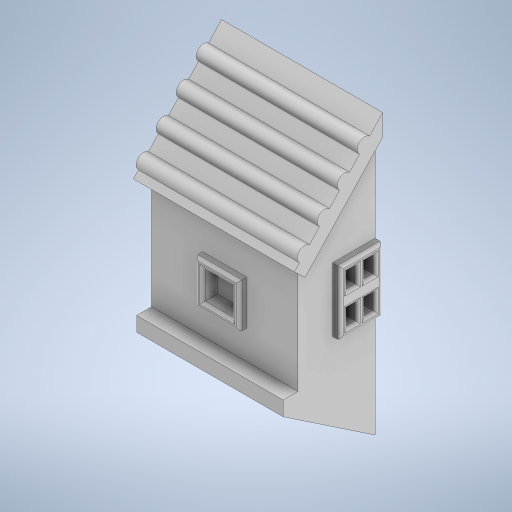
# Autodesk Inventor part: 背 物1
Saved by Autodesk Inventor 2024 (Build 280153000, 153)
## iProperties
Created: 2024-05-24
Part Number: 背 物1
Material: 一般
Document SubType Name: Modeling
Designer: User
Density: 1 g/cm^3
Appearance: 預設
Author: User
Autodesk Inventor part; units mm, degrees
ref_plane "YZ Plane" through (0, 0, 0) normal (1, 0, 0) x (0, 1, 0)
ref_plane "XZ Plane" through (0, 0, 0) normal (0, 1, 0) x (-1, 0, 0)
sketch "草圖1" plane through (0, 0, 0) normal (1, 0, 0) x (0, 1, 0)
  line L0 (0, 0) -> (7, 0)
  line L1 (7, 0) -> (7.6846, 0.7289)
  line L2 (7.6846, 0.7289) -> (14.0989, -5.2958)
  line L3 (0, 0) -> (0, 1)
  line L4 (0, 1) -> (-1, 1)
  line L5 (-1, 1) -> (-5.2258, -5.2958)
  line L6 (-5.2258, -5.2958) -> (14.0989, -5.2958)
  line L7 (7, 0) -> (12.6382, -5.2958)
  line L8 (2.0488, -5.2958) -> (6.4059, -5.2958)
  line L9 (6.4059, -5.2958) -> (6.4059, -2.3941)
  line L10 (6.4059, -2.3941) -> (2.0488, -2.3941)
  line L11 (2.0488, -2.3941) -> (2.0488, -5.2958)
  line L12 (5.9059, -2.8941) -> (4.7273, -2.8941)
  line L13 (4.7273, -2.8941) -> (4.7273, -3.5949)
  line L14 (4.7273, -3.5949) -> (5.9059, -3.5949)
  line L15 (5.9059, -3.5949) -> (5.9059, -2.8941)
  line L16 (4.7273, -4.0949) -> (5.9059, -4.0949)
  line L17 (5.9059, -4.0949) -> (5.9059, -4.7958)
  line L18 (5.9059, -4.7958) -> (4.7273, -4.7958)
  line L19 (4.7273, -4.7958) -> (4.7273, -4.0949)
  line L20 (3.7273, -2.8941) -> (2.5488, -2.8941)
  line L21 (2.5488, -2.8941) -> (2.5488, -3.5949)
  line L22 (2.5488, -3.5949) -> (3.7273, -3.5949)
  line L23 (3.7273, -3.5949) -> (3.7273, -2.8941)
  line L24 (3.7273, -4.0949) -> (2.5488, -4.0949)
  line L25 (2.5488, -4.0949) -> (2.5488, -4.7958)
  line L26 (2.5488, -4.7958) -> (3.7273, -4.7958)
  line L27 (3.7273, -4.7958) -> (3.7273, -4.0949)
  dimension "d0" = 7
  dimension "d1" = 1
  dimension "d2" = 8.8
  dimension "d3" = 1
  dimension "d4" = 1
  dimension "d5" = 0.5
  dimension "d6" = 0.5
  dimension "d7" = 0.5
  dimension "d8" = 0.5
  dimension "d9" = 0.5
  dimension "d10" = 0.5
  dimension "d11" = 1
  constraints: 56 end point, 11 parallel, 8 perpendicular, 7 point on line, 6 horizontal, 3 equal length, 2 collinear, 1 vertical
  measures "d0" distance of L0.start L0.end
  measures "d1" distance of L0.end L1.end
  measures "d2" distance of L1.end L2.end
  measures "d3" distance of L0.start L3.end
  measures "d4" distance of L3.end L4.end
  measures "d5" distance between parallel lines of L10 L12
  measures "d6" distance between parallel lines of L6 L18
  measures "d7" distance between parallel lines of L10 L20
  measures "d8" distance between parallel lines of L11 L21
  measures "d9" distance between parallel lines of L9 L15
  measures "d10" distance between parallel lines of L16 L14
  measures "d11" distance between parallel lines of L27 L19
extrude "擠出1" add sketch "草圖1" against normal blind 10 contours L0 L7 L6 L9 L10 L11 L5 L4 L3 | L6 L11 L10 L9 | L15 L14 L13 L12 | L16 L17 L18 L19 | L23 L22 L21 L20 | L27 L26 L25 L24
extrude "擠出2" add sketch "草圖1" along normal blind 0.5 and the other way blind 10.5 contours L1 L2 L6 L7
extrude "擠出3" add sketch "草圖1" along normal blind 0.5 contours L6 L11 L10 L9
extrude "擠出4" cut sketch "草圖1" against normal blind 0.5 contours L15 L14 L13 L12 | L16 L17 L18 L19 | L23 L22 L21 L20 | L27 L26 L25 L24
fillet "圓角1" radius 0.2 20 edges at (0.5, 6.4059, -3.8449) (0.5, 4.2273, -2.3941) (0.5, 2.0488, -3.8449) (0.5, 4.2273, -5.2958) (0.5, 5.3166, -2.8941) (0.5, 5.9059, -3.2445) (0.5, 5.3166, -3.5949) (0.5, 4.7273, -3.2445) (0.5, 3.7273, -3.2445) (0.5, 3.138, -3.5949) (0.5, 3.138, -2.8941) (0.5, 2.5488, -3.2445) (0.5, 2.5488, -4.4454) (0.5, 3.138, -4.0949) (0.5, 3.7273, -4.4454) (0.5, 3.138, -4.7958) (0.5, 5.3166, -4.7958) (0.5, 4.7273, -4.4454) (0.5, 5.3166, -4.0949) (0.5, 5.9059, -4.4454)
ref_plane "工作平面1" through (-5, 0, 0) normal (-1, 0, 0) x (0, 0, 1)
mirror "鏡射1" about plane through (-5, 0, 0) normal (-1, 0, 0) of "擠出3", "圓角1", "擠出4"
sketch "草圖2" plane through (-10, 0, 0) normal (0, 0, 1) x (1, 0, 0)
  line L0 (10, 7) -> (0, 7) projected
  line L1 (5, 7) -> (5, 0)
  line L2 (10, 0) -> (0, 0) projected
  line L3 (4, 2.5) -> (6, 2.5)
  line L4 (6, 2.5) -> (6, 4.5)
  line L5 (6, 4.5) -> (4, 4.5)
  line L6 (4, 4.5) -> (4, 2.5)
  line L7 (4, 2.5) -> (6, 4.5) construction
  line L8 (6, 2.5) -> (4, 4.5) construction
  line L9 (3.5, 2) -> (6.5, 2)
  line L10 (6.5, 2) -> (6.5, 5)
  line L11 (6.5, 5) -> (3.5, 5)
  line L12 (3.5, 5) -> (3.5, 2)
  line L13 (3.5, 2) -> (6.5, 5) construction
  line L14 (6.5, 2) -> (3.5, 5) construction
  point P0 (5, 3.5)
  point P1 (5, 3.5)
  dimension "d23" = 2
  dimension "d24" = 2
  dimension "d25" = 3
  dimension "d26" = 3
  constraints: 26 end point, 8 midpoint, 4 parallel, 2 horizontal, 2 perpendicular
  measures "d23" distance of L5.end L4.end
  measures "d24" distance of L4.end L3.end
  measures "d25" distance of L11.end L10.end
  measures "d26" distance of L10.end L9.end
extrude "擠出5" cut sketch "草圖2" against normal blind 0.5 contours L5 L4 L3 L1 | L1 L3 L6 L5
extrude "擠出6" add sketch "草圖2" along normal blind 0.5 contours L11 L10 L9 L1 L3 L4 L5 | L1 L5 L6 L3 L9 L12 L11
fillet "圓角2" radius 0.2 8 edges at (-5, 5, 0.5) (-3.5, 3.5, 0.5) (-6.5, 3.5, 0.5) (-5, 2, 0.5) (-5, 2.5, 0.5) (-4, 3.5, 0.5) (-5, 4.5, 0.5) (-6, 3.5, 0.5)
sketch "草圖3" plane through (0, -1, 1) normal (0, 0, 1) x (1, 0, 0)
  line L0 (0, 0) -> (-10, 0) projected
  line L1 (-8.3, 0) -> (-6.3, 0)
  line L2 (-6.3, 0) -> (-6.3, -5)
  line L3 (-6.3, -5) -> (-8.3, -5)
  line L4 (-8.3, -5) -> (-8.3, 0)
  line L5 (-3.7, 0) -> (-1.7, 0)
  line L6 (-1.7, 0) -> (-1.7, -5)
  line L7 (-1.7, -5) -> (-3.7, -5)
  line L8 (-3.7, -5) -> (-3.7, 0)
  line L9 (-10, -4.2258) -> (-10, 0) projected
  line L10 (0, 0) -> (0, -4.2258) projected
  point P0 (0, 1)
  point P1 (-1.7, 0)
  point P2 (-6.3, 0)
  dimension "d32" = 2
  dimension "d33" = 5
  dimension "d34" = 2
  dimension "d35" = 5
  dimension "d36" = 1.7
  dimension "d37" = 1.7
  constraints: 16 end point, 4 parallel, 2 horizontal, 2 perpendicular, 2 point on line
  measures "d32" distance of L2.end L3.end
  measures "d33" distance of L1.end L2.end
  measures "d34" distance of L6.end L7.end
  measures "d35" distance of L5.end L6.end
  measures "d36" distance between parallel lines of L9 L4
  measures "d37" distance between parallel lines of L10 L6
extrude "擠出7" cut sketch "草圖3" against normal up to surface (6.2958 mm away)
sketch "草圖4" plane through (0.5, 0, 0) normal (1, 0, 0) x (0, 0, -1)
  line L0 (-0.7289, 7.6846) -> (5.2958, 14.0989) projected
  arc A0 (0.298, 8.778) -> (-0.3866, 8.0491) centre (-0.0443, 8.4135) ccw
  arc A1 (1.6673, 10.2358) -> (0.9827, 9.5069) centre (1.325, 9.8713) ccw
  arc A2 (3.0366, 11.6935) -> (2.3519, 10.9646) centre (2.6942, 11.3291) ccw
  arc A3 (4.4058, 13.1513) -> (3.7212, 12.4224) centre (4.0635, 12.7869) ccw
  point P0 (0, 0)
  point P1 (4.4058, 13.1513)
  point P2 (3.7212, 12.4224)
  point P3 (2.3519, 10.9646)
  point P4 (1.6673, 10.2358)
  point P5 (0.9827, 9.5069)
  point P6 (0.298, 8.778)
  point P7 (-0.3866, 8.0491)
  dimension "d40" = 1.5
  dimension "d41" = 0.5
  dimension "d44" = 2
  constraints: 8 point on circle, 4 centre point, 1 other
  measures "d40" distance of L0.start A0.start
  measures "d41" radius of A0
  measures "d44" distance of A0.centre A1.centre
extrude "擠出8" add sketch "草圖4" against normal up to surface (11 mm away)
